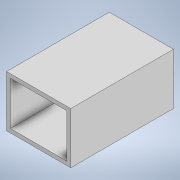
# Autodesk Inventor part: enclosure_80x40x50_mm
Saved by Autodesk Inventor 2020.2 (Build 242310000, 310)
## iProperties
Created: 2020-09-26
Part Number: enclosure_80x40x50_mm
Material: Generic
Document SubType Name: Modeling
Designer: Krishna Makhija
Density: 1 g/cm^3
Appearance: Default
Author: Krishna Makhija
Autodesk Inventor part; units mm, degrees
ref_plane "YZ Plane" through (0, 0, 0) normal (1, 0, 0) x (0, 1, 0)
ref_plane "XZ Plane" through (0, 0, 0) normal (0, 1, 0) x (-1, 0, 0)
ref_plane "XY Plane" through (0, 0, 0) normal (0, 0, 1) x (1, 0, 0)
sketch "Sketch1" plane through (0, 0, 0) normal (0, 0, 1) x (1, 0, 0)
  point P0 (0, 0)
sketch "Sketch2" plane through (0, 0, 0) normal (0, 0, 1) x (1, 0, 0)
  line L0 (22, -17) -> (-22, -17)
  line L1 (-22, -17) -> (-22, 17)
  line L2 (-22, 17) -> (22, 17)
  line L3 (22, 17) -> (22, -17)
  line L4 (22, -17) -> (-22, 17) construction
  line L5 (-22, -17) -> (22, 17) construction
  line L6 (25.0001, -20) -> (-25.0001, -20)
  line L7 (-25.0001, -20) -> (-25.0001, 20)
  line L8 (-25.0001, 20) -> (25.0001, 20)
  line L9 (25.0001, 20) -> (25.0001, -20)
  line L10 (25.0001, -20) -> (-25.0001, 20) construction
  line L11 (-25.0001, -20) -> (25.0001, 20) construction
  point P0 (0, 0)
  constraints: 24 end point, 4 midpoint, 4 parallel, 2 horizontal, 2 perpendicular
extrude "Extrusion1" add sketch "Sketch2" along normal blind 80
body "Solid1"
